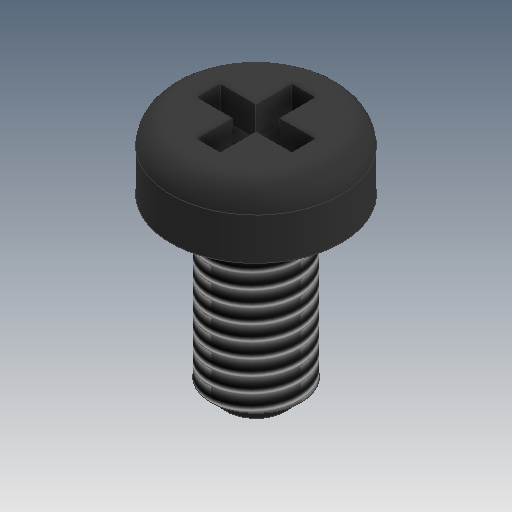
# Autodesk Inventor part: support_screw
Saved by Autodesk Inventor 2020 (Build 240168000, 168)
## iProperties
Created: 2020-10-02
Part Number: support_screw
Material: Generic
Document SubType Name: Modeling
Designer: DELL
Density: 1 g/cm^3
Appearance: Rubber - Black
Mass: 0.089304 g
Surface Area: 1.48375 cm^2
Volume: 0.089304 cm^3
Author: DELL
Autodesk Inventor part; units mm, degrees
ref_plane "YZ Plane" through (0, 0, 0) normal (1, 0, 0) x (0, 1, 0)
ref_plane "XZ Plane" through (0, 0, 0) normal (0, 1, 0) x (-1, 0, 0)
ref_plane "XY Plane" through (0, 0, 0) normal (0, 0, 1) x (1, 0, 0)
sketch "Sketch1" plane through (0, 0, 0) normal (0, 1, 0) x (-1, 0, 0)
  circle A0 centre (0, 0) radius 2.85
  dimension "d0" = 5.7
  constraints: 1 centre point, 1 coincident
  measures "d0" diameter of A0
extrude "Extrusion1" add sketch "Sketch1" along normal blind 2.2
sketch "Sketch2" plane through (0, 0, 0) normal (0, -1, 0) x (1, 0, 0)
  circle A0 centre (0, 0) radius 1.5
  dimension "d3" = 3
  constraints: 1 centre point, 1 coincident
  measures "d3" diameter of A0
extrude "Extrusion2" add sketch "Sketch2" along normal blind 5.8
fillet "Fillet1" radius 0.8 1 edges at (2.85, 2.2, 0)
sketch "Sketch3" plane through (0, 2.2, 0) normal (0, 1, 0) x (1, 0, 0)
  line L0 (0.4, -1.6) -> (-0.4, -1.6)
  line L1 (-0.4, -1.6) -> (-0.4, 1.6)
  line L2 (-0.4, 1.6) -> (0.4, 1.6)
  line L3 (0.4, 1.6) -> (0.4, -1.6)
  line L4 (0.4, -1.6) -> (-0.4, 1.6) construction
  line L5 (-0.4, -1.6) -> (0.4, 1.6) construction
  line L6 (1.6, 0.4) -> (-1.6, 0.4)
  line L7 (-1.6, 0.4) -> (-1.6, -0.4)
  line L8 (-1.6, -0.4) -> (1.6, -0.4)
  line L9 (1.6, -0.4) -> (1.6, 0.4)
  circle A0 centre (0, 0) radius 1.5 projected
  line L10 (1.6, 0.4) -> (-1.6, -0.4) construction
  line L11 (-1.6, 0.4) -> (1.6, -0.4) construction
  point P0 (0.4, 0.4)
  point P1 (-0.4, 0.4)
  point P2 (-0.4, -0.4)
  point P3 (0.4, -0.4)
  dimension "d7" = 0.8
  dimension "d8" = 0.8
  dimension "d9" = 3.2
  dimension "d10" = 3.2
  constraints: 24 end point, 4 midpoint, 4 parallel, 2 horizontal, 2 perpendicular
  measures "d7" distance of L1.end L2.end
  measures "d8" distance of L6.end L7.end
  measures "d9" distance of L2.end L0.start
  measures "d10" distance of L6.start L6.end
extrude "Extrusion3" cut sketch "Sketch3" against normal blind 1 contours L0 L1 A0 L3 | A0 L1 L8 L3 | L8 L1 L6 L3 | L3 L6 A0 L8 | A0 L6 L9 L8 | L8 A0 L6 L1 | L8 L7 L6 A0 | L6 L1 A0 L3 | A0 L1 L2 L3
chamfer "Chamfer1" distance 0.5 angle 45 1 edges at (-1.5, -5.8, 0)
thread "Thread1" size "M3x0.5" class "6g" standard "ANSI Metric M Profile" full length
body "Solid1"
